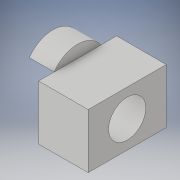
# Autodesk Inventor part: end peice for slides
Saved by Autodesk Inventor 2019 (Build 230136000, 136)
## iProperties
Created: 2019-05-04
Part Number: end peice for slides
Material: Generic
Document SubType Name: Modeling
Designer: User
Density: 1 g/cm^3
Appearance: Default
Author: User
Autodesk Inventor part; units mm, degrees
ref_plane "YZ Plane" through (0, 0, 0) normal (1, 0, 0) x (0, 1, 0)
ref_plane "XZ Plane" through (0, 0, 0) normal (0, 1, 0) x (-1, 0, 0)
ref_plane "XY Plane" through (0, 0, 0) normal (0, 0, 1) x (1, 0, 0)
sketch "Sketch1" plane through (0, 0, 0) normal (1, 0, 0) x (0, 1, 0)
  line L0 (0, 0) -> (7, 0)
  line L1 (7, 0) -> (7, -10)
  line L2 (7, -10) -> (0, -10)
  line L3 (0, -10) -> (0, 0)
  arc A0 (7, -8) -> (7, -2) centre (4.9527, -5) ccw
  point P0 (3.5, -5)
  dimension "d0" = 7
  dimension "d1" = 10
  dimension "d2" = 6
  dimension "d3" = 2
  constraints: 8 end point, 2 parallel, 2 point on circle, 2 point on line, 1 centre point, 1 horizontal, 1 perpendicular
  measures "d0" distance of L1.end L2.end
  measures "d1" distance of L0.end L1.end
  measures "d2" distance of A0.start A0.end
  measures "d3" distance of L1.end A0.start
extrude "Extrusion1" add sketch "Sketch1" along normal blind 6.35 contours L0 L1 L2 L3
extrude "Extrusion2" add sketch "Sketch1" against normal blind 3.175 contours A0 L1
sketch "Sketch2" plane through (0, 0, 0) normal (-1, 0, 0) x (0, 0, 1)
  line L0 (0, 0) -> (-10, 0) projected
  line L1 (0, 7) -> (0, 0) projected
  line L2 (-2, 7) -> (0, 7) projected
  line L3 (-8, 7) -> (-2, 7) projected
  line L4 (-10, 7) -> (-8, 7) projected
  line L5 (-10, 0) -> (-10, 7) projected
  circle A0 centre (-5, 3.5) radius 2.3812
  dimension "d15" = 4.7625
  constraints: 1 centre point, 1 coincident
  measures "d15" diameter of A0
extrude "Extrusion3" cut sketch "Sketch2" against normal through all contours A0
equation "\"d3\" = -0.5 * d2 + 0.5 * d1"
body "Solid1"
